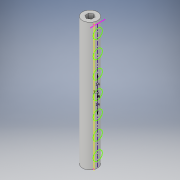
# Autodesk Inventor part: Spinner4inx12mm
Saved by Autodesk Inventor 2019 (Build 230136000, 136)
## iProperties
Created: 2018-09-29
Part Number: Spinner4inx12mm
Material: Generic
Document SubType Name: Modeling
Designer: mrhftc
Density: 1 g/cm^3
Appearance: Default
Author: mrhftc
Autodesk Inventor part; units mm, degrees
ref_plane "YZ Plane" through (0, 0, 0) normal (1, 0, 0) x (0, 1, 0)
sketch "Sketch3" plane through (0, 0, 0) normal (0, 1, 0) x (-1, 0, 0)
  circle A0 centre (0, 0) radius 6
  line L0 (0, 7.3639) -> (0, 0)
  line L1 (0, 0) -> (0, -8.8137)
  line L2 (6.485, 0) -> (0, 0)
  line L3 (-6.963, 0) -> (0, 0)
  line L4 (0, 3.0022) -> (2.6, 1.5011)
  line L5 (0, 3.0022) -> (3.0022, 3.0022) construction
  circle A1 centre (0, 0) radius 6
  line L6 (0, 3.0022) -> (-2.6, 1.5011)
  line L7 (0, -3.0022) -> (2.6, -1.5011)
  line L8 (0, -3.0022) -> (-2.6, -1.5011)
  line L9 (2.6, 1.5011) -> (2.6, -1.5011)
  line L10 (-2.6, 1.5011) -> (-2.6, -1.5011)
  dimension "d6" = 30
  dimension "d7" = 5.2
  dimension "d8" = 3.0022
  dimension "d9" = 3.0022
  dimension "d34" = 12
  constraints: 22 end point, 4 symmetric about line, 3 point on line, 2 centre point, 2 horizontal, 2 vertical, 1 coincident, 1 collinear, 1 equal length, 1 parallel, 1 other
  measures "d6" angle of L4 L5
  measures "d7" distance between parallel lines of L6 L7
  measures "d8" distance of L4.start L4.end
  measures "d9" distance of L4.end L7.end
  measures "d34" diameter of A0
extrude "Extrusion2" add sketch "Sketch3" along normal blind 101.6 contours L2 L9 L4 L0 A0 | A0 L1 L7 L9 L2 | L0 L6 L10 L3 A0 | A0 L3 L10 L8 L1
ref_plane "Work Plane1" through (0, 50.8, 0) normal (0, -1, 0) x (1, 0, 0)
ref_plane "Work Plane2" through (6, 0, 0) normal (-1, 0, 0) x (0, -1, 0)
sketch "Sketch4" plane through (6, 0, 0) normal (-1, 0, 0) x (0, -1, 0)
  line L0 (-99.6, 6) -> (-99.6, -6) projected
  line L1 (-99.6, 0) -> (0, 0)
  line L2 (0, 3.0022) -> (-101.6, 3.0022) projected
  circle A0 centre (-50.8, 0) radius 3.75
  circle A1 centre (-36.8, 0) radius 3.75
  circle A2 centre (-22.8, 0) radius 3.75
  circle A3 centre (-8.8, 0) radius 3.75
  circle A4 centre (-64.8, 0) radius 3.75
  circle A5 centre (-50.8, 0) radius 3.75
  circle A6 centre (-36.8, 0) radius 3.75
  circle A7 centre (-22.8, 0) radius 3.75
  circle A8 centre (-78.8, 0) radius 3.75
  circle A9 centre (-64.8, 0) radius 3.75
  circle A10 centre (-50.8, 0) radius 3.75
  circle A11 centre (-36.8, 0) radius 3.75
  circle A12 centre (-92.8, 0) radius 3.75
  circle A13 centre (-78.8, 0) radius 3.75
  circle A14 centre (-64.8, 0) radius 3.75
  circle A15 centre (-50.8, 0) radius 3.75
  point P0 (-1, 3.0022)
  point P1 (-100.6, 3.0022)
  dimension "d17" = 7.5
  dimension "d20" = 14
  dimension "d23" = 14
  constraints: 16 centre point, 2 end point, 2 horizontal, 1 parallel, 1 point on line, 30 other
  measures "d17" diameter of A0
  measures "d20" distance of A0.centre A1.centre
  measures "d23" distance of A0.centre A4.centre
sketch "Sketch5" plane through (0, 50.8, 0) normal (0, -1, 0) x (1, 0, 0)
  circle A0 centre (0, 0) radius 4
  dimension "d35" = 8
  constraints: 1 centre point, 1 coincident
  measures "d35" diameter of A0
extrude "Inner Cut" cut sketch "Sketch5" along normal mid plane 88.9
fillet "Inner hex fillets" radius 1 4 edges at (1.3, 6.35, -2.2517) (1.3, 6.35, 2.2517) (-1.3, 6.35, 2.2517) (-1.3, 6.35, -2.2517)
mirror "Mirror2" about plane through (0, 50.8, 0) normal (0, -1, 0) of "Inner hex fillets"
equation "\"d8\" = d9"
body "Solid2"
